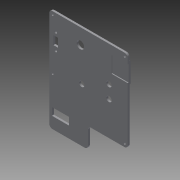
# Autodesk Inventor part: arduino-holder-cover
Saved by Autodesk Inventor 2014 (Build 180170000, 170)
## iProperties
Created: 2017-08-07
Part Number: arduino-holder-cover
Material: 一般
Document SubType Name: Modeling
Designer: hide
Density: 1 g/cm^3
Appearance: 既定
Author: hide
Autodesk Inventor part; units mm, degrees
ref_plane "YZ Plane" through (0, 0, 0) normal (1, 0, 0) x (0, 1, 0)
ref_plane "XZ Plane" through (0, 0, 0) normal (0, 1, 0) x (-1, 0, 0)
ref_plane "XY Plane" through (0, 0, 0) normal (0, 0, 1) x (1, 0, 0)
sketch "スケッチ5" plane through (0, 0, 0) normal (0, 1, 0) x (-1, 0, 0)
  line L0 (0, 0) -> (73, 0)
  line L1 (73, 0) -> (73, -76)
  line L2 (73, -76) -> (0, -76)
  line L3 (0, -76) -> (0, 0)
  line L4 (73, -76) -> (37, -76)
  line L5 (37, -76) -> (37, -95)
  line L6 (37, -95) -> (73, -95)
  line L7 (73, -95) -> (73, -76)
  line L8 (54.5, -84.5) -> (70.5, -84.5)
  line L9 (70.5, -84.5) -> (70.5, -77.5)
  line L10 (70.5, -77.5) -> (54.5, -77.5)
  line L11 (54.5, -77.5) -> (54.5, -84.5)
  circle A0 centre (17.5, -44.5) radius 2.5
  circle A1 centre (42.8, -45) radius 2.5
  circle A2 centre (44, -14.3) radius 3.5
  circle A3 centre (17.5, -32.5) radius 2.5
  line L12 (64.8943, -18.9476) -> (69.0943, -18.9476)
  line L13 (69.0943, -18.9476) -> (69.0943, -26.9476)
  line L14 (69.0943, -26.9476) -> (64.8943, -26.9476)
  line L15 (64.8943, -26.9476) -> (64.8943, -18.9476)
  circle A4 centre (66.9943, -15.4476) radius 1.2
  circle A5 centre (66.9943, -30.4476) radius 1.2
  line L16 (0, -8) -> (15, -8)
  line L17 (15, -8) -> (15, -23)
  line L18 (15, -23) -> (0, -23)
  line L19 (0, -23) -> (0, -8)
  dimension "d30" = 73
  dimension "d31" = 76
  dimension "d32" = 95
  dimension "d33" = 36
  dimension "d34" = 0
  dimension "d35" = 15
  dimension "d36" = 8
  dimension "d37" = 2.4
  dimension "d38" = 2.4
  dimension "d39" = 3.5
  dimension "d40" = 4.2
  dimension "d41" = 2.1
  dimension "d42" = 17.5
  dimension "d43" = 42.8
  dimension "d44" = 45
  dimension "d45" = 44.5
  dimension "d46" = 5
  dimension "d47" = 5
  dimension "d48" = 5
  dimension "d49" = 0
  dimension "d50" = 12
  dimension "d51" = 14.3
  dimension "d52" = 7
  dimension "d53" = 29
  dimension "d54" = 7
  dimension "d55" = 16
  dimension "d56" = 10.5
  dimension "d57" = 2.5
  dimension "d60" = 15
  dimension "d61" = 15
  dimension "d62" = 8
  constraints: 40 end point, 10 parallel, 6 centre point, 5 horizontal, 5 perpendicular, 1 point on line
  measures "d30" distance of L0.start L0.end
  measures "d31" distance of L2.end L0.start
  measures "d32" distance between parallel lines of L0 L6
  measures "d33" distance of L5.end L6.end
  measures "d34" horizontal distance of A5.centre A4.centre
  measures "d35" distance of A4.centre A5.centre
  measures "d36" distance of L14.end L12.start
  measures "d37" diameter of A4
  measures "d38" diameter of A5
  measures "d39" distance from line of L14 A5.centre
  measures "d40" distance of L12.start L12.end
  measures "d41" distance from line of A5.centre L15
  measures "d42" distance from line of A0.centre L3
  measures "d43" distance from line of L3 A1.centre
  measures "d44" distance from line of L0 A1.centre
  measures "d45" distance from line of L0 A0.centre
  measures "d46" diameter of A0
  measures "d47" diameter of A1
  measures "d48" diameter of A3
  measures "d49" horizontal distance of A0.centre A3.centre
  measures "d50" distance of A0.centre A3.centre
  measures "d51" distance from line of L0 A2.centre
  measures "d52" diameter of A2
  measures "d53" distance from line of L1 A2.centre
  measures "d54" distance of L8.end L9.end
  measures "d55" distance of L9.end L10.end
  measures "d56" distance between parallel lines of L6 L8
  measures "d57" distance between parallel lines of L7 L9
  measures "d60" distance of L16.start L16.end
  measures "d61" distance of L16.end L17.end
  measures "d62" distance between parallel lines of L0 L16
extrude "押し出し4" add sketch "スケッチ5" along normal blind 0.8 contours L0 L1 L2 L3 L18 L17 L16 | L7 L6 L5 L2
sketch "スケッチ6" plane through (0, 0.8, 0) normal (0, 1, 0) x (1, 0, 0)
  line L0 (0, 8) -> (-15, 8) projected
  line L1 (-15, 8) -> (-15, 23) projected
  line L2 (-15, 23) -> (0, 23) projected
  line L3 (0, 23) -> (0, 76) projected
  line L4 (0, 76) -> (-37, 76) projected
  line L5 (-37, 76) -> (-37, 95) projected
  line L6 (-37, 95) -> (-73, 95) projected
  line L7 (-73, 95) -> (-73, 0) projected
  line L8 (-73, 0) -> (0, 0) projected
  line L9 (0, 0) -> (0, 8) projected
  line L10 (-54.5, 84.5) -> (-54.5, 77.5) projected
  line L11 (-54.5, 77.5) -> (-70.5, 77.5) projected
  line L12 (-70.5, 77.5) -> (-70.5, 84.5) projected
  line L13 (-70.5, 84.5) -> (-54.5, 84.5) projected
  circle A0 centre (-66.9943, 15.4476) radius 1.2 projected
  circle A1 centre (-66.9943, 30.4476) radius 1.2 projected
  circle A2 centre (-17.5, 44.5) radius 2.5 projected
  circle A3 centre (-42.8, 45) radius 2.5 projected
  circle A4 centre (-17.5, 32.5) radius 2.5 projected
  line L14 (-69.0943, 18.9476) -> (-69.0943, 26.9476) projected
  line L15 (-69.0943, 26.9476) -> (-64.8943, 26.9476) projected
  line L16 (-64.8943, 26.9476) -> (-64.8943, 18.9476) projected
  line L17 (-64.8943, 18.9476) -> (-69.0943, 18.9476) projected
  circle A5 centre (-44, 14.3) radius 3.5 projected
  line L18 (0, 8) -> (-15, 8)
  line L19 (-15, 8) -> (-15, 23)
  line L20 (-15, 23) -> (0, 23)
  line L21 (0, 23) -> (0, 8)
  constraints: 8 end point, 2 parallel, 1 horizontal, 1 perpendicular
extrude "押し出し5" add sketch "スケッチ6" along normal blind 1
sketch "スケッチ7" plane through (0, 1.8, 0) normal (0, 1, 0) x (1, 0, 0)
  line L0 (0, 0) -> (0, 76) projected
  line L1 (0, 8) -> (-15, 8) projected
  line L2 (-15, 8) -> (-15, 23) projected
  line L3 (-15, 23) -> (0, 23) projected
  line L4 (0, 25) -> (-17, 25)
  line L5 (-17, 25) -> (-17, 6)
  line L6 (-17, 6) -> (0, 6)
  line L7 (0, 6) -> (0, 25)
  dimension "d65" = 2
  dimension "d66" = 2
  dimension "d67" = 2
  constraints: 8 end point, 2 parallel, 1 horizontal, 1 perpendicular, 1 point on line
  measures "d65" distance between parallel lines of L3 L4
  measures "d66" distance between parallel lines of L5 L2
  measures "d67" distance between parallel lines of L1 L6
extrude "押し出し6" add sketch "スケッチ7" along normal blind 1
fillet "フィレット3" radius 1 3 edges at (-8.5, 2.8, -25) (-17, 2.8, -15.5) (-8.5, 2.8, -6)
fillet "フィレット4" radius 3 6 edges at (-73, 0.9, 0) (0, 0.9, 0) (0, 0.9, -76) (-37, 0.9, -76) (-37, 0.9, -95) (-73, 0.9, -95)
sketch "スケッチ8" plane through (0, 1.8, 0) normal (0, 1, 0) x (1, 0, 0)
  line L0 (-73, 92) -> (-73, 3) projected
  line L1 (-70, 0) -> (-3, 0) projected
  line L2 (0, 3) -> (0, 6) projected
  line L3 (0, 25) -> (0, 73) projected
  line L4 (-3, 76) -> (-34, 76) projected
  circle A0 centre (-70, 3) radius 1
  circle A1 centre (-3, 3) radius 1
  circle A2 centre (-3, 73) radius 1
  circle A3 centre (-70, 50.5) radius 1
  point P0 (0, 0)
  dimension "d72" = 3
  dimension "d73" = 3
  dimension "d74" = 3
  dimension "d75" = 3
  dimension "d76" = 3
  dimension "d77" = 3
  dimension "d78" = 3
  dimension "d79" = 50.5
  dimension "d80" = 2
  dimension "d81" = 2
  dimension "d82" = 2
  dimension "d83" = 2
  constraints: 4 centre point
  measures "d72" distance from line of L0 A0.centre
  measures "d73" distance from line of L1 A0.centre
  measures "d74" distance from line of A1.centre L1
  measures "d75" distance from line of L2 A1.centre
  measures "d76" distance from line of L3 A2.centre
  measures "d77" distance from line of L4 A2.centre
  measures "d78" distance from line of L0 A3.centre
  measures "d79" distance from line of L1 A3.centre
  measures "d80" diameter of A3
  measures "d81" diameter of A0
  measures "d82" diameter of A2
  measures "d83" diameter of A1
extrude "押し出し7" cut sketch "スケッチ8" against normal blind 3
sketch "スケッチ9" plane through (0, 1.8, 0) normal (0, 1, 0) x (1, 0, 0)
  line L0 (-63.3045, 19.3424) -> (-56.9471, 19.3424) construction
  line L1 (-56.9471, 19.3424) -> (-56.9471, 16.216) construction
  line L2 (-56.9471, 16.216) -> (-63.3045, 16.216) construction
  line L3 (-63.3045, 16.216) -> (-63.3045, 19.3424) construction
  line L4 (-51.1909, 52.0748) -> (-37.3019, 52.0748) construction
  line L5 (-37.3019, 52.0748) -> (-37.3019, 49.0043) construction
  line L6 (-37.3019, 49.0043) -> (-51.1909, 49.0043) construction
  line L7 (-51.1909, 49.0043) -> (-51.1909, 52.0748) construction
  line L8 (-29.2834, 52.3325) -> (-5.2129, 52.3325) construction
  line L9 (-5.2129, 52.3325) -> (-5.2129, 43.6291) construction
  line L10 (-5.2129, 43.6291) -> (-29.2834, 43.6291) construction
  line L11 (-29.2834, 43.6291) -> (-29.2834, 52.3325) construction
  line L12 (-23.1622, 39.7679) -> (-12.0909, 39.7679) construction
  line L13 (-12.0909, 39.7679) -> (-12.0909, 36.7679) construction
  line L14 (-12.0909, 36.7679) -> (-23.1622, 36.7679) construction
  line L15 (-23.1622, 36.7679) -> (-23.1622, 39.7679) construction
  spline S0 degree 2 poles (-60.2632, 17.7792) (-60.2632, 17.0499) (-61.0411, 16.216) (-61.717, 16.216) knots 0 0 0 1 2 2 2
  spline S1 degree 2 poles (-61.717, 16.216) (-62.3953, 16.216) (-63.1683, 17.0596) (-63.1683, 17.7792) knots 0 0 0 1 2 2 2
  spline S2 degree 2 poles (-63.1683, 17.7792) (-63.1683, 18.5012) (-62.3953, 19.3424) (-61.717, 19.3424) knots 0 0 0 1 2 2 2
  spline S3 degree 2 poles (-61.717, 19.3424) (-61.0411, 19.3424) (-60.2632, 18.5061) (-60.2632, 17.7792) knots 0 0 0 1 2 2 2
  spline S4 degree 2 poles (-61.0411, 17.7792) (-61.0411, 18.049) (-61.1505, 18.4259) (-61.2453, 18.545) knots 0 0 0 1 2 2 2
  spline S5 degree 2 poles (-61.2453, 18.545) (-61.3401, 18.669) (-61.5833, 18.7759) (-61.7145, 18.7759) knots 0 0 0 1 2 2 2
  spline S6 degree 2 poles (-61.7145, 18.7759) (-61.8531, 18.7759) (-62.0792, 18.6763) (-62.1837, 18.5499) knots 0 0 0 1 2 2 2
  spline S7 degree 2 poles (-62.1837, 18.5499) (-62.2761, 18.4332) (-62.3904, 18.0466) (-62.3904, 17.7792) knots 0 0 0 1 2 2 2
  spline S8 degree 2 poles (-62.3904, 17.7792) (-62.3904, 17.502) (-62.281, 17.1374) (-62.1862, 17.0134) knots 0 0 0 1 2 2 2
  spline S9 degree 2 poles (-62.1862, 17.0134) (-62.0914, 16.8894) (-61.8458, 16.7824) (-61.7145, 16.7824) knots 0 0 0 1 2 2 2
  spline S10 degree 2 poles (-61.7145, 16.7824) (-61.5808, 16.7824) (-61.3329, 16.8967) (-61.2429, 17.0182) knots 0 0 0 1 2 2 2
  spline S11 degree 2 poles (-61.2429, 17.0182) (-61.1457, 17.1495) (-61.0411, 17.4972) (-61.0411, 17.7792) knots 0 0 0 1 2 2 2
  line L16 (-57.2461, 16.2792) -> (-57.9706, 16.2792)
  line L17 (-57.9706, 16.2792) -> (-59.1278, 18.3699)
  line L18 (-59.1278, 18.3699) -> (-59.1278, 16.2792)
  line L19 (-59.1278, 16.2792) -> (-59.8158, 16.2792)
  line L20 (-59.8158, 16.2792) -> (-59.8158, 19.2792)
  line L21 (-59.8158, 19.2792) -> (-58.892, 19.2792)
  line L22 (-58.892, 19.2792) -> (-57.9342, 17.5604)
  line L23 (-57.9342, 17.5604) -> (-57.9342, 19.2792)
  line L24 (-57.9342, 19.2792) -> (-57.2461, 19.2792)
  line L25 (-57.2461, 19.2792) -> (-57.2461, 16.2792)
  line L26 (-48.1083, 49.0116) -> (-49.0248, 49.0116)
  line L27 (-49.0248, 49.0116) -> (-49.8587, 50.1129)
  line L28 (-49.8587, 50.1129) -> (-50.131, 50.1129)
  line L29 (-50.131, 50.1129) -> (-50.131, 49.0116)
  line L30 (-50.131, 49.0116) -> (-50.8797, 49.0116)
  line L31 (-50.8797, 49.0116) -> (-50.8797, 52.0116)
  line L32 (-50.8797, 52.0116) -> (-49.6739, 52.0116)
  spline S12 degree 2 poles (-49.6739, 52.0116) (-49.4235, 52.0116) (-49.054, 51.9484) (-48.8959, 51.8511) knots 0 0 0 1 2 2 2
  spline S13 degree 2 poles (-48.8959, 51.8511) (-48.7355, 51.749) (-48.5459, 51.4306) (-48.5459, 51.1874) knots 0 0 0 1 2 2 2
  spline S14 degree 2 poles (-48.5459, 51.1874) (-48.5459, 50.8447) (-48.8571, 50.4144) (-49.1172, 50.2879) knots 0 0 0 1 2 2 2
  line L33 (-49.1172, 50.2879) -> (-48.1083, 49.0116)
  spline S15 degree 2 poles (-49.319, 51.0926) (-49.319, 51.2069) (-49.4065, 51.3698) (-49.5062, 51.4135) knots 0 0 0 1 2 2 2
  spline S16 degree 2 poles (-49.5062, 51.4135) (-49.5767, 51.4427) (-49.7493, 51.4597) (-49.8781, 51.4597) knots 0 0 0 1 2 2 2
  line L34 (-49.8781, 51.4597) -> (-50.131, 51.4597)
  line L35 (-50.131, 51.4597) -> (-50.131, 50.6526)
  line L36 (-50.131, 50.6526) -> (-49.9146, 50.6526)
  spline S17 degree 2 poles (-49.9146, 50.6526) (-49.759, 50.6526) (-49.5378, 50.6915) (-49.4624, 50.7523) knots 0 0 0 1 2 2 2
  spline S18 degree 2 poles (-49.4624, 50.7523) (-49.3895, 50.8106) (-49.319, 50.9662) (-49.319, 51.0926) knots 0 0 0 1 2 2 2
  spline S19 degree 2 poles (-45.1545, 50.5116) (-45.1545, 49.7823) (-45.9324, 48.9484) (-46.6083, 48.9484) knots 0 0 0 1 2 2 2
  spline S20 degree 2 poles (-46.6083, 48.9484) (-47.2865, 48.9484) (-48.0596, 49.792) (-48.0596, 50.5116) knots 0 0 0 1 2 2 2
  spline S21 degree 2 poles (-48.0596, 50.5116) (-48.0596, 51.2336) (-47.2865, 52.0748) (-46.6083, 52.0748) knots 0 0 0 1 2 2 2
  spline S22 degree 2 poles (-46.6083, 52.0748) (-45.9324, 52.0748) (-45.1545, 51.2385) (-45.1545, 50.5116) knots 0 0 0 1 2 2 2
  spline S23 degree 2 poles (-45.9324, 50.5116) (-45.9324, 50.7815) (-46.0418, 51.1583) (-46.1366, 51.2774) knots 0 0 0 1 2 2 2
  spline S24 degree 2 poles (-46.1366, 51.2774) (-46.2314, 51.4014) (-46.4746, 51.5084) (-46.6058, 51.5084) knots 0 0 0 1 2 2 2
  spline S25 degree 2 poles (-46.6058, 51.5084) (-46.7444, 51.5084) (-46.9705, 51.4087) (-47.075, 51.2823) knots 0 0 0 1 2 2 2
  spline S26 degree 2 poles (-47.075, 51.2823) (-47.1674, 51.1656) (-47.2817, 50.779) (-47.2817, 50.5116) knots 0 0 0 1 2 2 2
  spline S27 degree 2 poles (-47.2817, 50.5116) (-47.2817, 50.2344) (-47.1723, 49.8698) (-47.0775, 49.7458) knots 0 0 0 1 2 2 2
  spline S28 degree 2 poles (-47.0775, 49.7458) (-46.9827, 49.6218) (-46.7371, 49.5148) (-46.6058, 49.5148) knots 0 0 0 1 2 2 2
  spline S29 degree 2 poles (-46.6058, 49.5148) (-46.4721, 49.5148) (-46.2241, 49.6291) (-46.1342, 49.7507) knots 0 0 0 1 2 2 2
  spline S30 degree 2 poles (-46.1342, 49.7507) (-46.037, 49.8819) (-45.9324, 50.2296) (-45.9324, 50.5116) knots 0 0 0 1 2 2 2
  line L37 (-44.131, 49.0116) -> (-44.131, 51.4403)
  line L38 (-44.131, 51.4403) -> (-45.0183, 51.4403)
  line L39 (-45.0183, 51.4403) -> (-45.0183, 52.0116)
  line L40 (-45.0183, 52.0116) -> (-42.49, 52.0116)
  line L41 (-42.49, 52.0116) -> (-42.49, 51.4403)
  line L42 (-42.49, 51.4403) -> (-43.3773, 51.4403)
  line L43 (-43.3773, 51.4403) -> (-43.3773, 49.0116)
  line L44 (-43.3773, 49.0116) -> (-44.131, 49.0116)
  line L45 (-42.5045, 49.0116) -> (-41.4908, 52.0116)
  line L46 (-41.4908, 52.0116) -> (-40.669, 52.0116)
  line L47 (-40.669, 52.0116) -> (-39.6553, 49.0116)
  line L48 (-39.6553, 49.0116) -> (-40.4308, 49.0116)
  line L49 (-40.4308, 49.0116) -> (-40.618, 49.6242)
  line L50 (-40.618, 49.6242) -> (-41.5613, 49.6242)
  line L51 (-41.5613, 49.6242) -> (-41.7509, 49.0116)
  line L52 (-41.7509, 49.0116) -> (-42.5045, 49.0116)
  line L53 (-40.7833, 50.1688) -> (-41.0896, 51.1607)
  line L54 (-41.0896, 51.1607) -> (-41.3984, 50.1688)
  line L55 (-41.3984, 50.1688) -> (-40.7833, 50.1688)
  line L56 (-38.7801, 49.0116) -> (-38.7801, 51.4403)
  line L57 (-38.7801, 51.4403) -> (-39.6674, 51.4403)
  line L58 (-39.6674, 51.4403) -> (-39.6674, 52.0116)
  line L59 (-39.6674, 52.0116) -> (-37.1391, 52.0116)
  line L60 (-37.1391, 52.0116) -> (-37.1391, 51.4403)
  line L61 (-37.1391, 51.4403) -> (-38.0264, 51.4403)
  line L62 (-38.0264, 51.4403) -> (-38.0264, 49.0116)
  line L63 (-38.0264, 49.0116) -> (-38.7801, 49.0116)
  line L64 (-36.8303, 49.0116) -> (-36.8303, 52.0116)
  line L65 (-36.8303, 52.0116) -> (-34.8028, 52.0116)
  line L66 (-34.8028, 52.0116) -> (-34.8028, 51.4403)
  line L67 (-34.8028, 51.4403) -> (-36.0815, 51.4403)
  line L68 (-36.0815, 51.4403) -> (-36.0815, 50.9127)
  line L69 (-36.0815, 50.9127) -> (-34.9024, 50.9127)
  line L70 (-34.9024, 50.9127) -> (-34.9024, 50.3414)
  line L71 (-34.9024, 50.3414) -> (-36.0815, 50.3414)
  line L72 (-36.0815, 50.3414) -> (-36.0815, 49.5829)
  line L73 (-36.0815, 49.5829) -> (-34.8028, 49.5829)
  line L74 (-34.8028, 49.5829) -> (-34.8028, 49.0116)
  line L75 (-34.8028, 49.0116) -> (-36.8303, 49.0116)
  spline S31 degree 2 poles (-26.6651, 51.2531) (-26.6651, 51.044) (-26.7988, 50.6648) (-26.9228, 50.5384) knots 0 0 0 1 2 2 2
  spline S32 degree 2 poles (-26.9228, 50.5384) (-26.9982, 50.4581) (-27.1829, 50.3269) (-27.2923, 50.2807) knots 0 0 0 1 2 2 2
  spline S33 degree 2 poles (-27.2923, 50.2807) (-27.4042, 50.2345) (-27.6643, 50.181) (-27.8247, 50.181) knots 0 0 0 1 2 2 2
  line L76 (-27.8247, 50.181) -> (-28.2186, 50.181)
  line L77 (-28.2186, 50.181) -> (-28.2186, 49.1988)
  line L78 (-28.2186, 49.1988) -> (-28.9722, 49.1988)
  line L79 (-28.9722, 49.1988) -> (-28.9722, 52.1988)
  line L80 (-28.9722, 52.1988) -> (-27.8077, 52.1988)
  spline S34 degree 2 poles (-27.8077, 52.1988) (-27.55, 52.1988) (-27.1732, 52.104) (-27.02, 52.0019) knots 0 0 0 1 2 2 2
  spline S35 degree 2 poles (-27.02, 52.0019) (-26.8499, 51.8876) (-26.6651, 51.5133) (-26.6651, 51.2531) knots 0 0 0 1 2 2 2
  spline S36 degree 2 poles (-27.4382, 51.2337) (-27.4382, 51.3625) (-27.5597, 51.5449) (-27.6424, 51.5789) knots 0 0 0 1 2 2 2
  spline S37 degree 2 poles (-27.6424, 51.5789) (-27.7494, 51.6251) (-27.9439, 51.6397) (-28.1116, 51.6397) knots 0 0 0 1 2 2 2
  line L81 (-28.1116, 51.6397) -> (-28.2186, 51.6397)
  line L82 (-28.2186, 51.6397) -> (-28.2186, 50.7402)
  line L83 (-28.2186, 50.7402) -> (-28.1651, 50.7402)
  spline S38 degree 2 poles (-28.1651, 50.7402) (-28.0606, 50.7402) (-27.8709, 50.745) (-27.8004, 50.7572) knots 0 0 0 1 2 2 2
  spline S39 degree 2 poles (-27.8004, 50.7572) (-27.7396, 50.7669) (-27.6059, 50.8252) (-27.5695, 50.8617) knots 0 0 0 1 2 2 2
  spline S40 degree 2 poles (-27.5695, 50.8617) (-27.4917, 50.9346) (-27.4382, 51.0975) (-27.4382, 51.2337) knots 0 0 0 1 2 2 2
  line L84 (-24.2607, 49.1988) -> (-26.2615, 49.1988)
  line L85 (-26.2615, 49.1988) -> (-26.2615, 52.1988)
  line L86 (-26.2615, 52.1988) -> (-25.5079, 52.1988)
  line L87 (-25.5079, 52.1988) -> (-25.5079, 49.7701)
  line L88 (-25.5079, 49.7701) -> (-24.2607, 49.7701)
  line L89 (-24.2607, 49.7701) -> (-24.2607, 49.1988)
  line L90 (-24.2242, 49.1988) -> (-23.2105, 52.1988)
  line L91 (-23.2105, 52.1988) -> (-22.3888, 52.1988)
  line L92 (-22.3888, 52.1988) -> (-21.375, 49.1988)
  line L93 (-21.375, 49.1988) -> (-22.1505, 49.1988)
  line L94 (-22.1505, 49.1988) -> (-22.3377, 49.8115)
  line L95 (-22.3377, 49.8115) -> (-23.281, 49.8115)
  line L96 (-23.281, 49.8115) -> (-23.4706, 49.1988)
  line L97 (-23.4706, 49.1988) -> (-24.2242, 49.1988)
  line L98 (-22.503, 50.356) -> (-22.8093, 51.3479)
  line L99 (-22.8093, 51.3479) -> (-23.1181, 50.356)
  line L100 (-23.1181, 50.356) -> (-22.503, 50.356)
  line L101 (-18.5816, 52.1988) -> (-19.6173, 50.4509)
  line L102 (-19.6173, 50.4509) -> (-19.6173, 49.1988)
  line L103 (-19.6173, 49.1988) -> (-20.3709, 49.1988)
  line L104 (-20.3709, 49.1988) -> (-20.3709, 50.4144)
  line L105 (-20.3709, 50.4144) -> (-21.4236, 52.1988)
  line L106 (-21.4236, 52.1988) -> (-20.5654, 52.1988)
  line L107 (-20.5654, 52.1988) -> (-19.9795, 51.1291)
  line L108 (-19.9795, 51.1291) -> (-19.4131, 52.1988)
  line L109 (-19.4131, 52.1988) -> (-18.5816, 52.1988)
  line L110 (-16.61, 52.3325) -> (-17.8037, 48.5473)
  line L111 (-17.8037, 48.5473) -> (-18.3823, 48.5473)
  line L112 (-18.3823, 48.5473) -> (-17.191, 52.3325)
  line L113 (-17.191, 52.3325) -> (-16.61, 52.3325)
  spline S41 degree 2 poles (-15.003, 49.1453) (-15.3482, 49.1453) (-15.8685, 49.2791) (-16.0922, 49.3763) knots 0 0 0 1 2 2 2
  line L114 (-16.0922, 49.3763) -> (-16.0922, 50.091)
  line L115 (-16.0922, 50.091) -> (-16.0241, 50.091)
  spline S42 degree 2 poles (-16.0241, 50.091) (-15.798, 49.899) (-15.2559, 49.6923) (-15.0006, 49.6923) knots 0 0 0 1 2 2 2
  spline S43 degree 2 poles (-15.0006, 49.6923) (-14.9349, 49.6923) (-14.7234, 49.7215) (-14.6602, 49.7507) knots 0 0 0 1 2 2 2
  spline S44 degree 2 poles (-14.6602, 49.7507) (-14.5824, 49.7847) (-14.473, 49.9087) (-14.473, 50.0084) knots 0 0 0 1 2 2 2
  spline S45 degree 2 poles (-14.473, 50.0084) (-14.473, 50.1227) (-14.6505, 50.2637) (-14.7721, 50.2953) knots 0 0 0 1 2 2 2
  spline S46 degree 2 poles (-14.7721, 50.2953) (-14.9252, 50.3366) (-15.2729, 50.4071) (-15.426, 50.4606) knots 0 0 0 1 2 2 2
  spline S47 degree 2 poles (-15.426, 50.4606) (-15.7737, 50.5821) (-16.0751, 50.9979) (-16.0751, 51.309) knots 0 0 0 1 2 2 2
  spline S48 degree 2 poles (-16.0751, 51.309) (-16.0751, 51.7296) (-15.3628, 52.2523) (-14.828, 52.2523) knots 0 0 0 1 2 2 2
  spline S49 degree 2 poles (-14.828, 52.2523) (-14.5606, 52.2523) (-14.0306, 52.1429) (-13.8215, 52.0505) knots 0 0 0 1 2 2 2
  line L116 (-13.8215, 52.0505) -> (-13.8215, 51.365)
  line L117 (-13.8215, 51.365) -> (-13.8871, 51.365)
  spline S50 degree 2 poles (-13.8871, 51.365) (-14.0549, 51.5084) (-14.5362, 51.7053) (-14.7891, 51.7053) knots 0 0 0 1 2 2 2
  spline S51 degree 2 poles (-14.7891, 51.7053) (-14.8888, 51.7053) (-15.0443, 51.6761) (-15.1319, 51.6372) knots 0 0 0 1 2 2 2
  spline S52 degree 2 poles (-15.1319, 51.6372) (-15.2024, 51.6056) (-15.3045, 51.4792) (-15.3045, 51.4014) knots 0 0 0 1 2 2 2
  spline S53 degree 2 poles (-15.3045, 51.4014) (-15.3045, 51.2847) (-15.1416, 51.151) (-14.9082, 51.0975) knots 0 0 0 1 2 2 2
  spline S54 degree 2 poles (-14.9082, 51.0975) (-14.7575, 51.0635) (-14.4779, 50.9979) (-14.3174, 50.9419) knots 0 0 0 1 2 2 2
  spline S55 degree 2 poles (-14.3174, 50.9419) (-14.0063, 50.8277) (-13.7024, 50.4484) (-13.7024, 50.1372) knots 0 0 0 1 2 2 2
  spline S56 degree 2 poles (-13.7024, 50.1372) (-13.7024, 49.6899) (-14.405, 49.1453) (-15.003, 49.1453) knots 0 0 0 1 2 2 2
  line L118 (-12.7396, 49.1988) -> (-12.7396, 51.6275)
  line L119 (-12.7396, 51.6275) -> (-13.627, 51.6275)
  line L120 (-13.627, 51.6275) -> (-13.627, 52.1988)
  line L121 (-13.627, 52.1988) -> (-11.0986, 52.1988)
  line L122 (-11.0986, 52.1988) -> (-11.0986, 51.6275)
  line L123 (-11.0986, 51.6275) -> (-11.986, 51.6275)
  line L124 (-11.986, 51.6275) -> (-11.986, 49.1988)
  line L125 (-11.986, 49.1988) -> (-12.7396, 49.1988)
  spline S57 degree 2 poles (-8.0597, 50.6988) (-8.0597, 49.9695) (-8.8377, 49.1356) (-9.5136, 49.1356) knots 0 0 0 1 2 2 2
  spline S58 degree 2 poles (-9.5136, 49.1356) (-10.1918, 49.1356) (-10.9649, 49.9792) (-10.9649, 50.6988) knots 0 0 0 1 2 2 2
  spline S59 degree 2 poles (-10.9649, 50.6988) (-10.9649, 51.4209) (-10.1918, 52.262) (-9.5136, 52.262) knots 0 0 0 1 2 2 2
  spline S60 degree 2 poles (-9.5136, 52.262) (-8.8377, 52.262) (-8.0597, 51.4257) (-8.0597, 50.6988) knots 0 0 0 1 2 2 2
  spline S61 degree 2 poles (-8.8377, 50.6988) (-8.8377, 50.9687) (-8.9471, 51.3455) (-9.0419, 51.4646) knots 0 0 0 1 2 2 2
  spline S62 degree 2 poles (-9.0419, 51.4646) (-9.1367, 51.5886) (-9.3798, 51.6956) (-9.5111, 51.6956) knots 0 0 0 1 2 2 2
  spline S63 degree 2 poles (-9.5111, 51.6956) (-9.6497, 51.6956) (-9.8758, 51.5959) (-9.9803, 51.4695) knots 0 0 0 1 2 2 2
  spline S64 degree 2 poles (-9.9803, 51.4695) (-10.0727, 51.3528) (-10.187, 50.9663) (-10.187, 50.6988) knots 0 0 0 1 2 2 2
  spline S65 degree 2 poles (-10.187, 50.6988) (-10.187, 50.4217) (-10.0776, 50.057) (-9.9828, 49.933) knots 0 0 0 1 2 2 2
  spline S66 degree 2 poles (-9.9828, 49.933) (-9.8879, 49.809) (-9.6424, 49.7021) (-9.5111, 49.7021) knots 0 0 0 1 2 2 2
  spline S67 degree 2 poles (-9.5111, 49.7021) (-9.3774, 49.7021) (-9.1294, 49.8163) (-9.0395, 49.9379) knots 0 0 0 1 2 2 2
  spline S68 degree 2 poles (-9.0395, 49.9379) (-8.9422, 50.0692) (-8.8377, 50.4168) (-8.8377, 50.6988) knots 0 0 0 1 2 2 2
  spline S69 degree 2 poles (-5.3053, 51.2531) (-5.3053, 51.044) (-5.439, 50.6648) (-5.563, 50.5384) knots 0 0 0 1 2 2 2
  spline S70 degree 2 poles (-5.563, 50.5384) (-5.6383, 50.4581) (-5.8231, 50.3269) (-5.9325, 50.2807) knots 0 0 0 1 2 2 2
  spline S71 degree 2 poles (-5.9325, 50.2807) (-6.0443, 50.2345) (-6.3045, 50.181) (-6.4649, 50.181) knots 0 0 0 1 2 2 2
  line L126 (-6.4649, 50.181) -> (-6.8588, 50.181)
  line L127 (-6.8588, 50.181) -> (-6.8588, 49.1988)
  line L128 (-6.8588, 49.1988) -> (-7.6124, 49.1988)
  line L129 (-7.6124, 49.1988) -> (-7.6124, 52.1988)
  line L130 (-7.6124, 52.1988) -> (-6.4479, 52.1988)
  spline S72 degree 2 poles (-6.4479, 52.1988) (-6.1902, 52.1988) (-5.8134, 52.104) (-5.6602, 52.0019) knots 0 0 0 1 2 2 2
  spline S73 degree 2 poles (-5.6602, 52.0019) (-5.49, 51.8876) (-5.3053, 51.5133) (-5.3053, 51.2531) knots 0 0 0 1 2 2 2
  spline S74 degree 2 poles (-6.0784, 51.2337) (-6.0784, 51.3625) (-6.1999, 51.5449) (-6.2826, 51.5789) knots 0 0 0 1 2 2 2
  spline S75 degree 2 poles (-6.2826, 51.5789) (-6.3896, 51.6251) (-6.5841, 51.6397) (-6.7518, 51.6397) knots 0 0 0 1 2 2 2
  line L131 (-6.7518, 51.6397) -> (-6.8588, 51.6397)
  line L132 (-6.8588, 51.6397) -> (-6.8588, 50.7402)
  line L133 (-6.8588, 50.7402) -> (-6.8053, 50.7402)
  spline S76 degree 2 poles (-6.8053, 50.7402) (-6.7007, 50.7402) (-6.5111, 50.745) (-6.4406, 50.7572) knots 0 0 0 1 2 2 2
  spline S77 degree 2 poles (-6.4406, 50.7572) (-6.3798, 50.7669) (-6.2461, 50.8252) (-6.2097, 50.8617) knots 0 0 0 1 2 2 2
  spline S78 degree 2 poles (-6.2097, 50.8617) (-6.1319, 50.9346) (-6.0784, 51.0975) (-6.0784, 51.2337) knots 0 0 0 1 2 2 2
  line L134 (-20.2813, 36.7679) -> (-21.0058, 36.7679)
  line L135 (-21.0058, 36.7679) -> (-22.163, 38.8587)
  line L136 (-22.163, 38.8587) -> (-22.163, 36.7679)
  line L137 (-22.163, 36.7679) -> (-22.851, 36.7679)
  line L138 (-22.851, 36.7679) -> (-22.851, 39.7679)
  line L139 (-22.851, 39.7679) -> (-21.9272, 39.7679)
  line L140 (-21.9272, 39.7679) -> (-20.9693, 38.0491)
  line L141 (-20.9693, 38.0491) -> (-20.9693, 39.7679)
  line L142 (-20.9693, 39.7679) -> (-20.2813, 39.7679)
  line L143 (-20.2813, 39.7679) -> (-20.2813, 36.7679)
  line L144 (-19.6711, 36.7679) -> (-19.6711, 39.7679)
  line L145 (-19.6711, 39.7679) -> (-17.6435, 39.7679)
  line L146 (-17.6435, 39.7679) -> (-17.6435, 39.1966)
  line L147 (-17.6435, 39.1966) -> (-18.9223, 39.1966)
  line L148 (-18.9223, 39.1966) -> (-18.9223, 38.6691)
  line L149 (-18.9223, 38.6691) -> (-17.7432, 38.6691)
  line L150 (-17.7432, 38.6691) -> (-17.7432, 38.0978)
  line L151 (-17.7432, 38.0978) -> (-18.9223, 38.0978)
  line L152 (-18.9223, 38.0978) -> (-18.9223, 37.3392)
  line L153 (-18.9223, 37.3392) -> (-17.6435, 37.3392)
  line L154 (-17.6435, 37.3392) -> (-17.6435, 36.7679)
  line L155 (-17.6435, 36.7679) -> (-19.6711, 36.7679)
  line L156 (-14.5949, 36.7679) -> (-15.4653, 36.7679)
  line L157 (-15.4653, 36.7679) -> (-16.0439, 37.7234)
  line L158 (-16.0439, 37.7234) -> (-16.6346, 36.7679)
  line L159 (-16.6346, 36.7679) -> (-17.4685, 36.7679)
  line L160 (-17.4685, 36.7679) -> (-16.4936, 38.2777)
  line L161 (-16.4936, 38.2777) -> (-17.4296, 39.7679)
  line L162 (-17.4296, 39.7679) -> (-16.5593, 39.7679)
  line L163 (-16.5593, 39.7679) -> (-16.0171, 38.8611)
  line L164 (-16.0171, 38.8611) -> (-15.4604, 39.7679)
  line L165 (-15.4604, 39.7679) -> (-14.6265, 39.7679)
  line L166 (-14.6265, 39.7679) -> (-15.5674, 38.3093)
  line L167 (-15.5674, 38.3093) -> (-14.5949, 36.7679)
  line L168 (-13.7319, 36.7679) -> (-13.7319, 39.1966)
  line L169 (-13.7319, 39.1966) -> (-14.6192, 39.1966)
  line L170 (-14.6192, 39.1966) -> (-14.6192, 39.7679)
  line L171 (-14.6192, 39.7679) -> (-12.0909, 39.7679)
  line L172 (-12.0909, 39.7679) -> (-12.0909, 39.1966)
  line L173 (-12.0909, 39.1966) -> (-12.9782, 39.1966)
  line L174 (-12.9782, 39.1966) -> (-12.9782, 36.7679)
  line L175 (-12.9782, 36.7679) -> (-13.7319, 36.7679)
  point P0 (0, 0)
  constraints: 8 other
extrude "押し出し8" add sketch "スケッチ9" along normal blind 0.8
equation "\"d37\" = d38"
equation "\"d39\" = 0.5 * d35 - 0.5 * d36"
equation "\"d41\" = 0.5 * d40"
equation "\"d47\" = d46"
equation "\"d66\" = d65"
equation "\"d67\" = d65"
equation "\"d73\" = d72"
equation "\"d74\" = d73"
equation "\"d75\" = d72"
equation "\"d76\" = d72"
equation "\"d77\" = d76"
equation "\"d78\" = d72"
equation "\"d81\" = d80"
equation "\"d82\" = d80"
equation "\"d83\" = d80"
